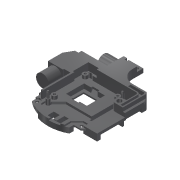
# Autodesk Inventor part: 01_XY_Actuator
Saved by Autodesk Inventor 2019 (Build 230136000, 136)
## iProperties
Created: 2018-09-04
Part Number: 01_XY_Actuator
Material: PC/ABS-Kunststoff
Document SubType Name: Modeling
Designer: Henry John
Density: 0.357273 g/cm^3
Appearance: Glatt - mittelgrau
Author: Henry John
Autodesk Inventor part; units mm, degrees
ref_plane "YZ Plane" through (0, 0, 0) normal (1, 0, 0) x (0, 1, 0)
ref_plane "XZ Plane" through (0, 0, 0) normal (0, 1, 0) x (-1, 0, 0)
ref_plane "XY Plane" through (0, 0, 0) normal (0, 0, 1) x (1, 0, 0)
sketch "Skizze1" plane through (0, 0, 0) normal (0, 0, 1) x (1, 0, 0)
  line L0 (-4.75, -3.625) -> (4.75, -3.625)
  line L1 (4.75, -3.625) -> (4.75, 3.625)
  line L2 (4.75, 3.625) -> (-4.75, 3.625)
  line L3 (-4.75, 3.625) -> (-4.75, -3.625)
  line L4 (-4.75, -3.625) -> (4.75, 3.625) construction
  line L5 (4.75, -3.625) -> (-4.75, 3.625) construction
  line L6 (13.75, -12.125) -> (13.75, 3.475)
  arc A0 (15.75, 5.475) -> (13.75, 3.475) centre (15.75, 3.475) ccw
  arc A1 (16.85, 5.475) -> (17.85, 6.475) centre (16.85, 6.475) ccw
  line L7 (17.85, 6.475) -> (17.85, 12.475)
  line L8 (17.85, 12.475) -> (19.45, 12.475)
  arc A2 (20.45, 11.475) -> (19.45, 12.475) centre (19.45, 11.475) ccw
  line L9 (20.45, 11.475) -> (20.45, 5.475)
  arc A3 (19.95, 4.975) -> (20.45, 5.475) centre (19.95, 5.475) ccw
  line L10 (19.95, 4.975) -> (18.7, 4.975)
  arc A4 (18.7, 4.975) -> (16.25, 2.525) centre (18.7, 2.525) ccw
  line L11 (16.25, 2.525) -> (16.25, -12.525)
  circle A5 centre (18.7, 2.525) radius 1.45
  line L12 (16.25, -12.525) -> (5.5, -12.525)
  line L13 (5.5, -12.525) -> (5.5, -12.125)
  line L14 (5.5, -12.125) -> (13.75, -12.125)
  circle A6 centre (-12.15, -18.0941) radius 0.9
  circle A7 centre (14.85, -17.225) radius 0.9
  line L15 (11.75, -19.125) -> (16.2, -19.125)
  line L16 (16.2, -19.125) -> (17.85, -17.475)
  line L17 (17.85, -17.475) -> (24.75, -17.475)
  line L18 (24.75, -17.475) -> (24.75, 12.025)
  line L19 (24.75, 12.025) -> (22.5561, 15.825)
  line L20 (22.5561, 15.825) -> (13.55, 15.825)
  line L21 (11.75, -19.125) -> (11.75, -21.875)
  line L22 (-14.25, -19.125) -> (-14.25, -13.625)
  line L23 (-15.45, -6.175) -> (-25.25, -6.175)
  line L24 (-25.25, -6.175) -> (-25.25, 10.825)
  line L25 (-25.25, 10.825) -> (-22.3632, 15.825)
  line L26 (-22.3632, 15.825) -> (-20.25, 15.825)
  line L27 (-12.25, 17.825) -> (-12.25, 28.125)
  line L28 (-12.25, 28.125) -> (-3.55, 28.125)
  line L29 (-3.55, 28.125) -> (-3.55, 30.625)
  line L30 (-3.55, 30.625) -> (5.55, 30.625)
  line L31 (5.55, 30.625) -> (5.55, 23.825)
  arc A8 (5.55, 23.825) -> (13.55, 15.825) centre (13.55, 23.825) ccw
  circle A9 centre (3.55, 28.625) radius 0.9
  line L32 (-20.25, 15.825) -> (-20.25, 17.825)
  line L33 (-20.25, 17.825) -> (-12.25, 17.825)
  line L34 (-14.25, -13.625) -> (-15.45, -13.625)
  line L35 (-15.45, -13.625) -> (-15.45, -6.175)
  line L36 (15.75, 5.475) -> (16.85, 5.475)
  arc A10 (-14.25, -19.125) -> (11.75, -21.875) centre (0.8733, -0.4247) ccw
  line L37 (30.6655, -24.475) -> (-37.4601, -24.475) construction
  point P0 (0, 0)
  dimension "d0" = 9.5
  dimension "d1" = 7.25
  dimension "d2" = 9
  dimension "d3" = 2
  dimension "d4" = 1
  dimension "d5" = 6
  dimension "d6" = 2.9
  dimension "d7" = 1
  dimension "d8" = 2.6
  dimension "d9" = 2.5
  dimension "d10" = 7.5
  dimension "d11" = 18
  dimension "d12" = 0.4
  dimension "d15" = 8.5
  dimension "d16" = 1.8
  dimension "d17" = 1.8
  dimension "d18" = 27
  dimension "d19" = 135
  dimension "d20" = 150
  dimension "d21" = 6.6
  dimension "d23" = 1.8
  dimension "d24" = 2
  dimension "d25" = 2
  dimension "d26" = 8
  dimension "d27" = 27
  dimension "d28" = 14.8
  dimension "d30" = 9.1
  dimension "d31" = 17.8
  dimension "d32" = 2.5
  dimension "d33" = 1
  dimension "d34" = 0.5
  dimension "d35" = 2.75
  dimension "d36" = 20
  dimension "d38" = 26
  dimension "d40" = 1.2
  dimension "d41" = 1
  dimension "d42" = 3
  dimension "d44" = 20
  dimension "d46" = 5.5
  dimension "d47" = 1.2
  dimension "d48" = 11
  dimension "d49" = 150
  dimension "d50" = 5
  dimension "d51" = 8
  dimension "d52" = 2
  dimension "d53" = 5
  dimension "d111" = 4.3
  dimension "d221" = 10.75
  dimension "d252" = 50
  dimension "d254" = 55.1
  dimension "d255" = 1.2
  dimension "d256" = 24
  dimension "d269" = 29.5
  constraints: 77 end point, 17 perpendicular, 14 point on circle, 13 tangent, 11 centre point, 6 parallel, 5 horizontal, 4 vertical, 2 midpoint, 1 coincident, 1 collinear, 1 point on line
  measures "d0" distance of L2.end L1.end
  measures "d1" distance of L1.end L0.end
  measures "d2" distance between parallel lines of L6 L1
  measures "d3" radius of A0
  measures "d4" radius of A1
  measures "d5" distance of L7.start L7.end
  measures "d6" diameter of A5
  measures "d7" radial gap between concentric circles of A4 A5
  measures "d8" distance between parallel lines of L9 L7
  measures "d9" distance between parallel lines of L6 L11
  measures "d10" distance between parallel lines of L8 L10
  measures "d11" distance from line of L12 L36.end
  measures "d12" distance between parallel lines of L14 L12
  measures "d15" distance between parallel lines of L14 L0
  measures "d16" diameter of A7
  measures "d17" diameter of A6
  measures "d18" horizontal distance of A7.centre A6.centre
  measures "d19" angle of L16 L15
  measures "d20" angle of L19 L18
  measures "d21" distance between parallel lines of L15 L12
  measures "d23" diameter of A9
  measures "d24" distance from line of A9.centre L30
  measures "d25" distance from line of L31 A9.centre
  measures "d26" radius of A8
  measures "d27" distance between parallel lines of L30 L2
  measures "d28" distance between parallel lines of L20 L30
  measures "d30" distance of L29.end L30.end
  measures "d31" distance between parallel lines of L27 L31
  measures "d32" distance of L28.end L29.end
  measures "d33" radius of A2
  measures "d34" radius of A3
  measures "d35" distance of L15.start L21.end
  measures "d36" distance from line of L17 A4.centre
  measures "d38" distance between parallel lines of L21 L22
  measures "d40" distance edge to line of A6 L22
  measures "d41" distance edge to line of A7 L15
  measures "d42" horizontal distance of A7.centre L16.end
  measures "d44" distance between parallel lines of L18 L1
  measures "d46" distance from line of L22.start L34
  measures "d47" distance between parallel lines of L35 L22
  measures "d48" distance between parallel lines of L24 L22
  measures "d49" angle of L24 L25
  measures "d50" distance from line of L24.end L26
  measures "d51" distance between parallel lines of L32 L27
  measures "d52" distance between parallel lines of L26 L33
  measures "d53" distance between parallel lines of L24 L32
  measures "d111" distance between parallel lines of L18 L9
  measures "d221" distance between parallel lines of L11 L13
  measures "d252" distance between parallel lines of L18 L24
  measures "d256" distance between parallel lines of L23 L33
  measures "d269" distance from line of L18.end L17
extrude "Extrusion1" add sketch "Skizze1" along normal blind 9
sketch "Skizze2" plane through (-25.25, -6.175, 0) normal (0, -1, 0) x (1, 0, 0)
  line L0 (0, 0) -> (9.8, 0) projected
  line L1 (9.8, 0) -> (9.8, 9) projected
  line L2 (0, 9) -> (9.8, 9) projected
  line L3 (0, 0) -> (0, 9) projected
  circle A0 centre (4.5, 4.5) radius 4.5 construction
  circle A1 centre (4.5, 4.5) radius 4
  point P0 (25.25, 0)
  dimension "d60" = 8
  constraints: 3 tangent, 2 centre point, 1 coincident
  measures "d60" diameter of A1
extrude "Extrusion2" cut sketch "Skizze2" against normal blind 8
sketch "Skizze3" plane through (-12.25, 17.825, 0) normal (-1, 0, 0) x (0, 0, 1)
  line L0 (0, 10.3) -> (0, 0) projected
  line L1 (0, 0) -> (9, 0) projected
  line L2 (9, 10.3) -> (9, 0) projected
  line L3 (0, 10.3) -> (9, 10.3) projected
  circle A0 centre (4.5, 5.8) radius 4.5 construction
  circle A1 centre (4.5, 5.8) radius 4
  point P0 (0, -17.825)
  dimension "d61" = 8
  constraints: 3 tangent, 2 centre point, 1 coincident
  measures "d61" diameter of A1
extrude "Extrusion3" cut sketch "Skizze3" against normal blind 8
sketch "Skizze4" plane through (0, 0, 9) normal (0, 0, 1) x (1, 0, 0)
  line L0 (-15.95, 2.525) -> (-11.95, 2.525)
  line L1 (-11.95, 2.525) -> (-11.95, -15.975)
  line L2 (-11.95, -15.975) -> (-10.95, -15.975)
  line L3 (-10.95, -15.975) -> (-10.95, 4.025)
  line L4 (-10.95, 4.025) -> (-11.95, 4.025)
  line L5 (-11.95, 4.025) -> (-11.95, 13.775)
  line L6 (-11.95, 13.775) -> (-5.45, 13.775)
  line L7 (-5.45, 13.775) -> (-5.45, 12.475)
  line L8 (-5.45, 12.475) -> (18.95, 12.475)
  line L9 (20.45, 10.975) -> (20.45, 6.725)
  arc A0 (18.7, 4.975) -> (20.45, 6.725) centre (18.7, 6.725) ccw
  arc A1 (18.7, 4.975) -> (16.25, 2.525) centre (18.7, 2.525) ccw
  line L10 (18.25, -0.025) -> (25.25, -0.025)
  line L11 (25.25, -0.025) -> (25.25, -25.475)
  line L12 (25.25, -25.475) -> (-15.95, -25.475)
  line L13 (-15.95, -25.475) -> (-15.95, 2.525)
  circle A2 centre (18.7, 2.525) radius 1.45 construction
  line L14 (20.45, 11.475) -> (20.45, 5.475) construction
  arc A3 (20.45, 10.975) -> (18.95, 12.475) centre (18.95, 10.975) ccw
  line L15 (17.85, 12.475) -> (19.45, 12.475) projected
  line L16 (-15.45, 1.825) -> (-15.45, -13.625) construction
  line L17 (24.75, -17.475) -> (24.75, 12.025) construction
  arc A4 (18.7, 4.975) -> (16.25, 2.525) centre (18.7, 2.525) ccw construction
  line L18 (16.25, 2.525) -> (16.25, 1.975)
  line L19 (16.25, 2.525) -> (16.25, -12.525) construction
  arc A5 (16.25, 1.975) -> (18.25, -0.025) centre (18.25, 1.975) ccw
  arc A6 (-14.25, -19.125) -> (11.75, -21.875) centre (0.8733, -0.4247) ccw construction
  point P0 (0, 0)
  dimension "d64" = 1.5
  dimension "d66" = 1.3
  dimension "d67" = 6.5
  dimension "d68" = 1
  dimension "d69" = 9.75
  dimension "d70" = 20
  dimension "d71" = 1
  dimension "d72" = 18.5
  dimension "d73" = 0.5
  dimension "d74" = 0.5
  dimension "d75" = 2
  dimension "d76" = 5
  dimension "d257" = 1
  dimension "d258" = 32.4
  constraints: 30 end point, 11 perpendicular, 8 point on circle, 4 centre point, 4 tangent, 2 collinear, 2 horizontal, 2 horizontal alignment, 2 point on line, 2 vertical alignment, 1 coincident, 1 concentric
  measures "d64" radius of A3
  measures "d66" distance between parallel lines of L8 L6
  measures "d67" distance of L5.end L6.end
  measures "d68" distance between parallel lines of L5 L3
  measures "d69" distance between parallel lines of L4 L6
  measures "d70" distance of L2.end L3.end
  measures "d71" distance of L1.end L2.end
  measures "d72" distance of L0.end L1.end
  measures "d73" distance between parallel lines of L16 L13
  measures "d74" distance between parallel lines of L17 L11
  measures "d75" radius of A5
  measures "d76" distance from line of A0.start L10
  measures "d257" distance edge to line of A6 L12
  measures "d258" distance between parallel lines of L5 L9
extrude "Extrusion4" cut sketch "Skizze4" against normal blind 4.7
sketch "Skizze5" plane through (0, 0, 4.3) normal (0, 0, 1) x (1, 0, 0)
  circle A0 centre (-12.15, -18.0941) radius 0.9 projected
  line L0 (-14.25, -13.625) -> (-14.25, -19.125) projected
  line L1 (-14.25, -16.8941) -> (-13.75, -16.8941)
  line L2 (-10.15, -18.0941) -> (-10.15, -21.8)
  line L3 (-10.15, -21.8) -> (-14.25, -21.8)
  line L4 (-14.25, -21.8) -> (-14.25, -16.8941)
  arc A1 (-10.15, -18.0941) -> (-13.75, -16.8941) centre (-12.15, -18.0941) ccw
  line L5 (9.75, -22.7769) -> (9.75, -18.7769)
  line L6 (9.75, -18.7769) -> (13.5519, -14.975)
  line L7 (13.5519, -14.975) -> (16.5519, -14.975)
  line L8 (16.5519, -14.975) -> (16.5519, -17.475)
  line L9 (16.5519, -17.475) -> (18.35, -17.475)
  line L10 (18.35, -17.475) -> (18.35, -22.7769)
  line L11 (18.35, -22.7769) -> (9.75, -22.7769)
  line L12 (24.75, -17.475) -> (17.85, -17.475) construction
  line L13 (11.75, -19.125) -> (11.75, -21.875) construction
  line L14 (7.75, -24.4681) -> (7.75, -16.8171)
  line L15 (7.75, -16.8171) -> (12.4421, -12.125)
  line L16 (13.75, -12.125) -> (13.75, -9.925)
  line L17 (13.75, 3.475) -> (13.75, -12.125) construction
  line L18 (13.75, -9.925) -> (-2.25, -9.925)
  line L19 (-4.75, -3.625) -> (4.75, -3.625) projected
  line L20 (-2.25, -9.925) -> (-6.7793, -14.4543)
  line L21 (-6.7793, -14.4543) -> (-6.7793, -15.4543)
  arc A2 (-9.15, -15.7181) -> (-6.7793, -15.4543) centre (-7.9793, -15.4543) ccw
  line L22 (-9.15, -15.7181) -> (-9.15, -18.4681)
  line L23 (-9.15, -18.4681) -> (-5.55, -22.0681)
  line L24 (-5.55, -22.0681) -> (-3.55, -22.0681)
  line L25 (-3.55, -22.0681) -> (-3.05, -22.5681)
  line L26 (-3.05, -22.5681) -> (-1.05, -22.5681)
  line L27 (-1.05, -22.5681) -> (-0.55, -23.0681)
  line L28 (-0.55, -23.0681) -> (1.45, -23.0681)
  line L29 (1.45, -23.0681) -> (1.45, -24.4681)
  line L30 (1.45, -24.4681) -> (7.75, -24.4681)
  line L31 (5.5, -12.525) -> (16.25, -12.525) construction
  arc A3 (-14.25, -19.125) -> (11.75, -21.875) centre (0.8733, -0.4247) ccw construction
  arc A4 (-14.25, -19.125) -> (11.75, -21.875) centre (0.8733, -0.4247) ccw construction
  line L32 (13.75, -12.125) -> (5.5, -12.125) projected
  line L33 (13.75, -12.125) -> (12.4421, -12.125)
  point P0 (0, 0)
  point P1 (0.2761, -24.4676)
  point P2 (1.4706, -24.4676)
  dimension "d79" = 2
  dimension "d80" = 0.5
  dimension "d81" = 4
  dimension "d82" = 135
  dimension "d83" = 2.5
  dimension "d84" = 3
  dimension "d85" = 2
  dimension "d86" = 0.5
  dimension "d87" = 2.6
  dimension "d90" = 2
  dimension "d91" = 6.3
  dimension "d92" = 1.4
  dimension "d93" = 2
  dimension "d94" = 0.5
  dimension "d95" = 2
  dimension "d96" = 0.5
  dimension "d97" = 2
  dimension "d98" = 1
  dimension "d99" = 1.2
  dimension "d100" = 1
  dimension "d104" = 2.75
  dimension "d105" = 16
  dimension "d280" = 2.8
  constraints: 54 end point, 8 parallel, 7 perpendicular, 7 point on circle, 5 horizontal, 4 collinear, 3 vertical, 2 centre point, 2 point on line, 2 tangent, 1 coincident
  measures "d79" radius of A1
  measures "d80" distance of L1.start L1.end
  measures "d81" distance of L5.start L5.end
  measures "d82" angle of L5 L6
  measures "d83" distance of L7.end L8.end
  measures "d84" distance of L6.end L7.end
  measures "d85" distance between parallel lines of L13 L5
  measures "d86" distance from line of L12.end L10
  measures "d87" distance between parallel lines of L31 L18
  measures "d90" distance between parallel lines of L14 L5
  measures "d91" distance between parallel lines of L29 L14
  measures "d92" distance of L28.end L29.end
  measures "d93" distance of L27.end L28.end
  measures "d94" distance between parallel lines of L26 L28
  measures "d95" distance of L25.end L26.end
  measures "d96" distance between parallel lines of L26 L24
  measures "d97" distance of L23.end L24.end
  measures "d98" distance between parallel lines of L22 L2
  measures "d99" radius of A2
  measures "d100" distance of L20.end L21.end
  measures "d104" distance of L22.start L22.end
  measures "d105" distance of L16.end L18.end
  measures "d280" distance between parallel lines of L6 L15
extrude "Extrusion5" cut sketch "Skizze5" against normal blind 1
sketch "Skizze6" plane through (0, 0, 9) normal (0, 0, 1) x (1, 0, 0)
  line L0 (23.35, 14.4499) -> (24.75, 14.4499)
  line L1 (24.75, 14.4499) -> (24.75, -0.025)
  line L2 (24.75, -0.025) -> (23.35, -0.025)
  line L3 (23.35, -0.025) -> (23.35, 14.4499)
  line L4 (20.45, 11.475) -> (20.45, 5.475) construction
  line L5 (24.75, -0.025) -> (24.75, 12.025) construction
  line L6 (24.75, 12.025) -> (22.5561, 15.825) construction
  line L7 (18.25, -0.025) -> (24.75, -0.025) construction
  line L8 (21.15, 0.775) -> (22.55, 0.775)
  line L9 (22.55, 0.775) -> (22.55, 13.8355)
  line L10 (22.55, 13.8355) -> (21.9787, 14.825)
  line L11 (21.9787, 14.825) -> (13.45, 14.825)
  line L12 (13.45, 14.825) -> (13.45, 13.175)
  line L13 (13.45, 13.175) -> (19.45, 13.175)
  arc A0 (21.15, 11.475) -> (19.45, 13.175) centre (19.45, 11.475) ccw
  line L14 (21.15, 11.475) -> (21.15, 0.775)
  arc A1 (20.45, 11.475) -> (19.45, 12.475) centre (19.45, 11.475) ccw construction
  circle A2 centre (18.7, 2.525) radius 1.45 construction
  line L15 (22.5561, 15.825) -> (13.55, 15.825) construction
  point P0 (0, 0)
  dimension "d110" = 2.9
  dimension "d112" = 0.8
  dimension "d113" = 1
  dimension "d114" = 1
  dimension "d115" = 1
  dimension "d116" = 0.8
  dimension "d117" = 7
  constraints: 22 end point, 4 parallel, 4 perpendicular, 2 collinear, 2 horizontal, 2 point on circle, 2 tangent, 1 centre point, 1 concentric, 1 point on line, 1 vertical
  measures "d110" distance between parallel lines of L4 L3
  measures "d112" distance between parallel lines of L7 L8
  measures "d113" distance edge to line of A2 L14
  measures "d114" distance between parallel lines of L15 L11
  measures "d115" distance between parallel lines of L6 L10
  measures "d116" distance between parallel lines of L3 L9
  measures "d117" distance between parallel lines of L12 L4
extrude "Extrusion6" cut sketch "Skizze6" against normal blind 2.3
sketch "Skizze7" plane through (0, 0, 4.3) normal (0, 0, 1) x (1, 0, 0)
  circle A0 centre (-7.9793, -15.4543) radius 1.2
  arc A1 (-9.15, -15.7181) -> (-6.7793, -15.4543) centre (-7.9793, -15.4543) ccw construction
  circle A2 centre (-7.9793, -11.4543) radius 1.575
  circle A3 centre (-7.9793, -11.4543) radius 0.7
  circle A4 centre (-9.45, 9.3) radius 1.575
  circle A5 centre (-9.45, 9.3) radius 0.7
  circle A6 centre (12.7, 7.475) radius 1.575
  circle A7 centre (12.7, 7.475) radius 0.7
  line L0 (-5.45, 12.475) -> (19.45, 12.475) construction
  circle A8 centre (15.7, 7.475) radius 0.75
  line L1 (-11.95, 4.025) -> (-11.95, 13.775) projected
  line L2 (20.45, 11.475) -> (20.45, 5.475) construction
  line L3 (-11.95, 13.775) -> (-5.45, 13.775) construction
  point P0 (0, 0)
  dimension "d120" = 3.15
  dimension "d121" = 1.4
  dimension "d122" = 4
  dimension "d123" = 3.15
  dimension "d124" = 1.4
  dimension "d127" = 3.15
  dimension "d128" = 1.4
  dimension "d130" = 5
  dimension "d132" = 1.5
  dimension "d281" = 2.5
  dimension "d282" = 4
  dimension "d283" = 3
  dimension "d284" = 2.9
  constraints: 8 centre point, 3 coincident, 2 concentric, 1 horizontal alignment, 1 vertical alignment
  measures "d120" diameter of A2
  measures "d121" diameter of A3
  measures "d122" distance of A2.centre A0.centre
  measures "d123" diameter of A4
  measures "d124" diameter of A5
  measures "d127" diameter of A6
  measures "d128" diameter of A7
  measures "d130" distance from line of A6.centre L0
  measures "d132" diameter of A8
  measures "d281" distance from line of L1 A4.centre
  measures "d282" distance edge to line of A8 L2
  measures "d283" distance of A8.centre A6.centre
  measures "d284" distance edge to line of A4 L3
extrude "Extrusion7" add sketch "Skizze7" along normal blind 2
sketch "Skizze8" plane through (-7.9793, -15.4543, 6.3) normal (0, 0, 1) x (1, 0, 0)
  circle A0 centre (0, 0) radius 1.2 construction
  circle A1 centre (23.6793, 22.9293) radius 0.75 projected
  circle A2 centre (0, 0) radius 0.75
  point P0 (7.9793, 15.4543)
  dimension "d135" = 1.5
  constraints: 1 centre point, 1 coincident
  measures "d135" diameter of A2
extrude "Extrusion8" add sketch "Skizze8" along normal blind 4
sketch "Skizze9" plane through (0, 0, 9) normal (0, 0, 1) x (1, 0, 0)
  line L0 (-3.55, 30.625) -> (-3.55, 28.125) projected
  line L1 (-3.55, 28.125) -> (-2.05, 28.125)
  line L2 (-2.05, 28.125) -> (-2.05, 26.625)
  line L3 (-2.05, 26.625) -> (5.55, 26.625)
  line L4 (5.55, 26.625) -> (5.55, 30.625)
  line L5 (5.55, 30.625) -> (-3.55, 30.625) projected
  line L6 (5.55, 30.625) -> (-3.55, 30.625)
  line L7 (-3.55, 30.625) -> (-3.55, 28.125)
  point P0 (0, 0)
  dimension "d138" = 1.5
  constraints: 12 end point, 5 perpendicular, 1 collinear, 1 horizontal
  measures "d138" distance of L0.end L1.end
extrude "Extrusion9" cut sketch "Skizze9" against normal blind 3
sketch "Skizze10" plane through (0, 0, 0) normal (0, 0, -1) x (-1, 0, 0)
  line L0 (2.05, 26.625) -> (2.05, 28.125) projected
  line L1 (2.05, 28.125) -> (3.55, 28.125) projected
  line L2 (3.55, 28.125) -> (3.55, 30.625) projected
  line L3 (3.55, 30.625) -> (-5.55, 30.625) projected
  line L4 (2.05, 26.625) -> (2.05, 15.925)
  line L5 (2.05, 15.925) -> (1.55, 15.925)
  line L6 (0.55, 18.925) -> (0.55, 24.625)
  line L7 (0.55, 24.625) -> (-2.45, 24.625)
  line L8 (-2.45, 24.625) -> (-2.45, 19.625)
  line L9 (-2.45, 19.625) -> (-3.45, 19.625)
  arc A0 (-8.55, 15.825) -> (-3.45, 19.625) centre (-10.386, 23.6115) ccw
  line L10 (-8.55, 15.825) -> (-13.55, 15.825)
  arc A1 (-13.55, 15.825) -> (-5.55, 23.825) centre (-13.55, 23.825) ccw projected
  arc A2 (-13.55, 15.825) -> (-5.55, 23.825) centre (-13.55, 23.825) ccw projected
  line L11 (-5.55, 23.825) -> (-5.55, 30.625) projected
  arc A3 (-13.55, 15.825) -> (-5.55, 23.825) centre (-13.55, 23.825) ccw projected
  line L12 (-0.45, 23.625) -> (-1.45, 23.625)
  line L13 (-1.45, 23.625) -> (-1.45, 18.625)
  line L14 (-1.45, 18.625) -> (-2.8937, 18.625)
  arc A4 (-5.7043, 15.925) -> (-2.8937, 18.625) centre (-10.386, 23.6115) ccw
  line L15 (-5.7043, 15.925) -> (0.4959, 15.925)
  line L16 (0.4959, 15.925) -> (-0.45, 18.7627)
  line L17 (-0.45, 18.7627) -> (-0.45, 23.625)
  line L18 (1.55, 15.925) -> (0.55, 18.925)
  point P0 (0, 0)
  dimension "d141" = 5
  dimension "d142" = 1
  dimension "d143" = 3
  dimension "d144" = 1.5
  dimension "d145" = 14.7
  dimension "d146" = 6
  dimension "d147" = 11
  dimension "d148" = 3
  dimension "d149" = 1
  dimension "d150" = 1
  dimension "d151" = 1
  dimension "d152" = 1
  dimension "d153" = 1
  dimension "d154" = 1
  dimension "d155" = 1
  constraints: 28 end point, 7 perpendicular, 5 point on circle, 3 horizontal, 2 centre point, 2 vertical, 1 collinear, 1 concentric, 1 equal radius, 1 parallel
  measures "d141" distance of L10.start L10.end
  measures "d142" distance of L8.end L9.end
  measures "d143" distance of L6.end L7.end
  measures "d144" distance between parallel lines of L4 L6
  measures "d145" distance between parallel lines of L3 L5
  measures "d146" distance between parallel lines of L3 L7
  measures "d147" distance between parallel lines of L9 L3
  measures "d148" distance from line of L6.start L5
  measures "d149" distance from line of L5.end L6
  measures "d150" distance between parallel lines of L17 L6
  measures "d151" distance between parallel lines of L8 L13
  measures "d152" distance between parallel lines of L7 L12
  measures "d153" distance between parallel lines of L18 L16
  measures "d154" radial gap between concentric circles of A0 A4
  measures "d155" distance between parallel lines of L9 L14
extrude "Extrusion10" cut sketch "Skizze10" against normal blind 3.5
sketch "Skizze12" plane through (0, 0, 0) normal (0, 0, -1) x (-1, 0, 0)
  line L0 (-17.85, -17.475) -> (-16.2, -17.475)
  line L1 (-16.2, -17.475) -> (-16.2, -14.125)
  line L2 (-16.2, -14.125) -> (-7.6, -14.125)
  line L3 (-7.6, -14.125) -> (-7.6, -19.125)
  line L4 (-7.6, -19.125) -> (-16.2, -19.125)
  line L5 (-16.2, -19.125) -> (-17.85, -17.475)
  circle A0 centre (-9.6, -16.625) radius 0.75
  point P0 (0, 0)
  dimension "d165" = 5
  dimension "d166" = 8.6
  dimension "d167" = 1.5
  dimension "d168" = 2.5
  dimension "d169" = 2
  constraints: 12 end point, 4 perpendicular, 2 coincident, 1 centre point, 1 horizontal, 1 point on line
  measures "d165" distance between parallel lines of L4 L2
  measures "d166" distance between parallel lines of L3 L1
  measures "d167" diameter of A0
  measures "d168" distance from line of A0.centre L4
  measures "d169" distance from line of L3 A0.centre
extrude "Extrusion12" cut sketch "Skizze12" against normal blind 2.5
chamfer "Fase1" distance 0.25 distance2 1 1 edges at (10.35, -16.625, 0) measured on face at (9.85, -16.625, 0)
chamfer "Fase2" distance 0.25 distance2 1 1 edges at (-8.7293, -15.4543, 10.3) measured on face at (-8.2293, -15.4543, 10.3)
chamfer "Fase3" distance 0.25 distance2 1 1 edges at (14.95, 7.475, 10.3) measured on face at (15.45, 7.475, 10.3)
sketch "Skizze11" plane through (0, 0, 0) normal (0, 0, -1) x (-1, 0, 0)
  line L0 (6.45, -23.3329) -> (6.45, -18.125)
  line L1 (6.45, -18.125) -> (9.5, -18.125)
  line L2 (9.5, -18.125) -> (9.5, -14.625)
  line L3 (9.5, -14.625) -> (10.5, -13.625)
  line L4 (10.5, -13.625) -> (15.45, -13.625)
  line L5 (15.45, -13.625) -> (15.45, -23.3329)
  line L6 (15.45, -23.3329) -> (6.45, -23.3329)
  line L7 (15.45, -13.625) -> (14.25, -13.625) construction
  line L8 (15.45, -13.625) -> (15.45, 1.825) construction
  line L9 (14.25, -13.625) -> (14.25, -19.125) projected
  arc A0 (-11.75, -21.875) -> (14.25, -19.125) centre (-0.8733, -0.4247) ccw construction
  point P0 (0, 0)
  dimension "d158" = 135
  dimension "d160" = 1
  dimension "d161" = 4.5
  dimension "d162" = 9
  dimension "d223" = 4.75
  constraints: 14 end point, 3 perpendicular, 2 collinear, 1 horizontal, 1 parallel, 1 point on circle, 1 vertical
  measures "d158" angle of L2 L3
  measures "d160" distance from line of L2.end L4
  measures "d161" distance between parallel lines of L4 L1
  measures "d162" distance between parallel lines of L0 L5
  measures "d223" distance between parallel lines of L2 L9
extrude "Extrusion11" cut sketch "Skizze11" against normal blind 2.3
sketch "Skizze13" plane through (0, 0, 0) normal (0, 0, -1) x (-1, 0, 0)
  line L0 (6.95, 6.15) -> (-3.8, 6.15)
  line L1 (-3.8, 6.15) -> (-3.8, 7.65)
  arc A0 (-3.8, 7.65) -> (-6.2, 7.65) centre (-5, 7.65) ccw
  line L2 (-6.2, 7.65) -> (-6.2, 6.15)
  line L3 (-6.2, 6.15) -> (-6.95, 6.15)
  line L4 (-6.95, 6.15) -> (-6.95, -6.15)
  line L5 (-6.95, -6.15) -> (3.75, -6.15)
  line L6 (3.75, -6.15) -> (3.75, -7.65)
  arc A1 (3.75, -7.65) -> (6.15, -7.65) centre (4.95, -7.65) ccw
  line L7 (6.15, -7.65) -> (6.15, -6.15)
  line L8 (6.15, -6.15) -> (6.95, -6.15)
  line L9 (6.95, -6.15) -> (6.95, 6.15)
  line L10 (3.25, -6.65) -> (3.25, -8.1)
  arc A2 (3.25, -8.1) -> (4.25, -9.1) centre (4.25, -8.1) ccw
  line L11 (4.25, -9.1) -> (6.45, -9.1)
  arc A3 (6.45, -9.1) -> (7.45, -8.1) centre (6.45, -8.1) ccw
  line L12 (7.45, -8.1) -> (7.45, 9.15)
  line L13 (7.45, 9.15) -> (-3.25, 9.15)
  line L14 (-3.25, 9.15) -> (-3.25, 10.65)
  arc A4 (-3.25, 10.65) -> (-4.25, 11.65) centre (-4.25, 10.65) ccw
  line L15 (-4.25, 11.65) -> (-6.75, 11.65)
  arc A5 (-6.75, 11.65) -> (-7.75, 10.65) centre (-6.75, 10.65) ccw
  line L16 (-7.75, 10.65) -> (-7.75, -6.65)
  line L17 (-7.75, -6.65) -> (3.25, -6.65)
  line L18 (6.95, 6.15) -> (-6.95, -6.15) construction
  line L19 (6.95, -6.15) -> (-6.95, 6.15) construction
  circle A6 centre (4.95, -7.65) radius 0.45
  circle A7 centre (-5, 7.65) radius 0.45
  line L20 (1.7, -21.525) -> (1.7, -18.325)
  line L21 (6.45, -18.125) -> (-2.05, -18.125)
  line L22 (-2.05, -18.125) -> (-2.05, -22.125)
  line L23 (-2.05, -22.125) -> (-4.05, -22.125)
  line L24 (-4.05, -22.125) -> (-4.05, -13.575)
  line L25 (-4.05, -13.575) -> (-5.5, -12.125)
  line L26 (-5.5, -12.125) -> (-9.8, -12.125)
  line L27 (-9.8, -12.125) -> (-9.8, -12.525)
  line L28 (-9.8, -12.525) -> (-7.8, -12.525)
  line L29 (-7.8, -12.525) -> (-6.8, -13.525)
  line L30 (-6.8, -13.525) -> (-6.8, -20.025)
  line L31 (-6.8, -20.025) -> (-8.3, -20.025)
  line L32 (-8.3, -20.025) -> (-8.3, -21.525)
  line L33 (-8.3, -21.525) -> (-6.8, -21.525)
  arc A8 (-6.8, -21.525) -> (-5.8, -22.525) centre (-5.8, -21.525) ccw
  line L34 (-5.8, -22.525) -> (0.7, -22.525)
  arc A9 (0.7, -22.525) -> (1.7, -21.525) centre (0.7, -21.525) ccw
  line L35 (-5.5, -12.525) -> (-16.25, -12.525) construction
  line L36 (-13.75, -12.125) -> (-5.5, -12.125) construction
  line L37 (-7.6, -14.125) -> (-7.6, -19.125) construction
  line L38 (-16.25, -12.525) -> (-16.25, 2.525) construction
  line L39 (-7.6, -19.125) -> (-11.75, -19.125) construction
  line L40 (9.5, -18.125) -> (9.5, -14.625) construction
  line L41 (6.45, -18.125) -> (9.5, -18.125) construction
  line L42 (1.7, -18.325) -> (6.45, -18.325)
  line L43 (6.45, -18.325) -> (6.45, -18.125)
  point P0 (0, 0)
  point P1 (0, 0)
  point P2 (0, 0)
  dimension "d181" = 15.2
  dimension "d182" = 15.8
  dimension "d183" = 4.5
  dimension "d184" = 1
  dimension "d185" = 3
  dimension "d186" = 0.5
  dimension "d187" = 2.4
  dimension "d188" = 1.5
  dimension "d189" = 0.8
  dimension "d190" = 0.5
  dimension "d191" = 2
  dimension "d193" = 2.4
  dimension "d195" = 4.2
  dimension "d196" = 18.25
  dimension "d197" = 1.5
  dimension "d198" = 18.3
  dimension "d199" = 2.75
  dimension "d202" = 0.9
  dimension "d203" = 0.9
  dimension "d207" = 0.8
  dimension "d210" = 1
  dimension "d211" = 0.9
  dimension "d212" = 1.5
  dimension "d213" = 1
  dimension "d214" = 8.5
  dimension "d219" = 0.4
  dimension "d224" = 0.2
  dimension "d225" = 45
  dimension "d230" = 1.5
  dimension "d231" = 2
  dimension "d232" = 2.75
  dimension "d233" = 2
  constraints: 74 end point, 22 perpendicular, 16 point on circle, 14 tangent, 10 centre point, 6 point on line, 4 equal radius, 4 horizontal, 3 coincident, 3 parallel, 2 collinear, 2 midpoint, 2 vertical, 1 vertical alignment
  measures "d181" distance between parallel lines of L16 L12
  measures "d182" distance between parallel lines of L13 L17
  measures "d183" distance between parallel lines of L16 L14
  measures "d184" radius of A4
  measures "d185" distance between parallel lines of L13 L0
  measures "d186" distance between parallel lines of L5 L17
  measures "d187" distance between parallel lines of L2 L1
  measures "d188" distance from line of L0 A0.centre
  measures "d189" distance between parallel lines of L16 L4
  measures "d190" distance between parallel lines of L12 L9
  measures "d191" distance from line of L9 A1.centre
  measures "d193" distance between parallel lines of L6 L7
  measures "d195" distance between parallel lines of L10 L12
  measures "d196" distance between parallel lines of L13 L11
  measures "d197" distance from line of L5 A1.centre
  measures "d198" distance between parallel lines of L17 L15
  measures "d199" distance from line of L16 A0.centre
  measures "d202" diameter of A6
  measures "d203" diameter of A7
  measures "d207" distance between parallel lines of L30 L37
  measures "d210" distance from line of L28 L29.end
  measures "d211" distance between parallel lines of L39 L31
  measures "d212" distance of L30.end L31.end
  measures "d213" radius of A8
  measures "d214" distance between parallel lines of L20 L30
  measures "d219" distance between parallel lines of L34 L23
  measures "d224" distance between parallel lines of L21 L42
  measures "d225" angle of L30 L29
  measures "d230" distance between parallel lines of L31 L33
  measures "d231" distance from line of L28.end L27
  measures "d232" distance between parallel lines of L30 L24
  measures "d233" distance between parallel lines of L22 L24
extrude "Extrusion13" cut sketch "Skizze13" against normal blind 2
sketch "Skizze14" plane through (0, 0, 0) normal (0, 0, -1) x (-1, 0, 0)
  line L0 (4.75, 3.625) -> (4.75, -3.625) projected
  line L1 (4.75, -3.625) -> (-4.75, -3.625) projected
  line L2 (-4.75, -3.625) -> (-4.75, 3.625) projected
  line L3 (-4.75, 3.625) -> (4.75, 3.625) projected
  circle A0 centre (-5, 7.65) radius 0.45 projected
  line L4 (-3.8, 6.15) -> (-3.8, 7.65) projected
  arc A1 (-3.8, 7.65) -> (-6.2, 7.65) centre (-5, 7.65) ccw projected
  line L5 (-6.2, 7.65) -> (-6.2, 6.15) projected
  line L6 (-6.2, 6.15) -> (-6.95, 6.15) projected
  line L7 (-6.95, 6.15) -> (-6.95, -6.15) projected
  line L8 (-6.95, -6.15) -> (3.75, -6.15) projected
  line L9 (3.75, -6.15) -> (3.75, -7.65) projected
  arc A2 (3.75, -7.65) -> (6.15, -7.65) centre (4.95, -7.65) ccw projected
  line L10 (6.15, -7.65) -> (6.15, -6.15) projected
  line L11 (6.15, -6.15) -> (6.95, -6.15) projected
  line L12 (6.95, -6.15) -> (6.95, 6.15) projected
  line L13 (6.95, 6.15) -> (-3.8, 6.15) projected
  circle A3 centre (4.95, -7.65) radius 0.45 projected
extrude "Extrusion14" cut sketch "Skizze14" against normal blind 0.5
sketch "Skizze15" plane through (0, 0, 2) normal (0, 0, -1) x (-1, 0, 0)
  arc A0 (-3.25, 10.65) -> (-4.25, 11.65) centre (-4.25, 10.65) ccw projected
  line L0 (-6.75, 11.65) -> (-4.25, 11.65) projected
  arc A1 (-6.75, 11.65) -> (-7.75, 10.65) centre (-6.75, 10.65) ccw projected
  line L1 (-3.25, 9.85) -> (-7.75, 9.85)
  line L2 (-7.75, 10.65) -> (-7.75, 9.85)
  line L3 (-3.25, 10.65) -> (-3.25, 9.85)
  line L4 (1.7, -18.325) -> (1.7, -21.525) projected
  arc A2 (0.7, -22.525) -> (1.7, -21.525) centre (0.7, -21.525) ccw projected
  line L5 (0.7, -22.525) -> (-5.8, -22.525) projected
  arc A3 (-6.8, -21.525) -> (-5.8, -22.525) centre (-5.8, -21.525) ccw projected
  line L6 (-2.05, -22.125) -> (-2.05, -18.125) projected
  line L7 (-4.05, -22.125) -> (-2.05, -22.125) projected
  line L8 (-4.05, -22.125) -> (-4.05, -17.225)
  line L9 (-4.05, -17.225) -> (-6.8, -17.225)
  line L10 (-6.8, -17.225) -> (-6.8, -21.525)
  line L11 (-2.05, -18.125) -> (1.7, -18.125)
  line L12 (1.7, -18.125) -> (1.7, -18.325)
  point P0 (0, 0)
  dimension "d226" = 1.8
  dimension "d227" = 5.3
  constraints: 16 end point, 3 perpendicular, 3 vertical, 2 horizontal
  measures "d226" distance between parallel lines of L0 L1
  measures "d227" distance between parallel lines of L9 L5
extrude "Extrusion15" cut sketch "Skizze15" along normal through all both and the other way through all
sketch "Skizze16" plane through (0, 0, 4.3) normal (0, 0, 1) x (1, 0, 0)
  line L0 (-6.5, 5.625) -> (-6.5, -5.625)
  line L1 (6.5, -5.625) -> (6.5, 5.625)
  line L2 (-2.1, 5.625) -> (-2.1, 6.65)
  line L3 (-2.1, 6.65) -> (2.1, 6.65)
  line L4 (2.1, 6.65) -> (2.1, 5.625)
  line L5 (2.1, -5.625) -> (2.1, -6.65)
  line L6 (2.1, -6.65) -> (-2.1, -6.65)
  line L7 (-2.1, -6.65) -> (-2.1, -5.625)
  line L8 (-6.5, -5.625) -> (-2.1, -5.625)
  line L9 (2.1, -5.625) -> (6.5, -5.625)
  line L10 (6.5, 5.625) -> (2.1, 5.625)
  line L11 (-2.1, 5.625) -> (-6.5, 5.625)
  line L12 (-6.5, -5.625) -> (6.5, 5.625) construction
  line L13 (-6.5, 5.625) -> (6.5, -5.625) construction
  line L14 (-2.1, 6.65) -> (2.1, -6.65) construction
  line L15 (-2.1, -6.65) -> (2.1, 6.65) construction
  point P0 (0, 0)
  point P1 (0, 0)
  point P2 (0, -6.65)
  dimension "d234" = 4.2
  dimension "d235" = 13
  dimension "d236" = 11.25
  dimension "d237" = 13.3
  constraints: 32 end point, 6 perpendicular, 5 parallel, 4 midpoint, 4 point on line, 2 collinear, 2 horizontal, 1 coincident, 1 vertical, 1 vertical alignment
  measures "d234" distance between parallel lines of L7 L5
  measures "d235" distance between parallel lines of L0 L1
  measures "d236" distance between parallel lines of L9 L10
  measures "d237" distance between parallel lines of L6 L3
extrude "Extrusion16" cut sketch "Skizze16" against normal blind 2.9
sketch "Skizze17" plane through (0, 0, 3.3) normal (0, 0, 1) x (1, 0, 0)
  arc A0 (-9.1793, -15.4543) -> (-7.6793, -16.9543) centre (-7.6793, -15.4543) ccw
  arc A1 (-6.4509, -16.9543) -> (-4.9509, -15.4543) centre (-6.4509, -15.4543) ccw
  line L0 (-7.6793, -16.9543) -> (-6.4509, -16.9543)
  line L1 (-4.9509, -15.4543) -> (-2.0216, -12.525)
  line L2 (-2.0216, -12.525) -> (13.75, -12.525)
  line L3 (13.75, -9.925) -> (-2.25, -9.925)
  line L4 (-2.25, -9.925) -> (-6.7793, -14.4543)
  line L5 (-6.7793, -14.4543) -> (-6.7793, -15.4543)
  line L6 (-2.25, -9.925) -> (13.75, -9.925) construction
  line L7 (5.5, -12.525) -> (12.0421, -12.525) construction
  line L8 (-6.7793, -14.4543) -> (-2.25, -9.925) construction
  line L9 (-6.7793, -15.4543) -> (-6.7793, -14.4543) construction
  circle A2 centre (-7.9793, -15.4543) radius 1.2 construction
  arc A3 (-9.1793, -15.4543) -> (-6.7793, -15.4543) centre (-7.9793, -15.4543) ccw
  line L10 (13.75, -9.925) -> (13.75, -12.525)
  line L11 (13.75, 3.475) -> (13.75, -12.125) construction
  point P0 (0, 0)
  point P1 (13.5714, -9.925)
  dimension "d241" = 1.5
  dimension "d243" = 2
  constraints: 14 end point, 7 point on circle, 4 collinear, 4 horizontal alignment, 4 point on line, 3 centre point, 3 tangent, 2 horizontal, 1 concentric, 1 parallel, 1 perpendicular
  measures "d241" radius of A1
  measures "d243" distance between parallel lines of L1 L4
extrude "Extrusion17" cut sketch "Skizze17" against normal blind 0.4
sketch "Skizze18" plane through (0, 0, 4.3) normal (0, 0, 1) x (1, 0, 0)
  line L0 (7.75, 9.85) -> (3.25, 9.85) projected
  line L1 (7.75, 9.85) -> (15.85, 9.85)
  arc A0 (17.85, 7.85) -> (15.85, 9.85) centre (15.85, 7.85) ccw
  line L2 (17.85, 12.475) -> (17.85, 6.475) construction
  line L3 (17.85, 7.85) -> (17.85, 6.475)
  line L4 (17.85, 6.475) -> (18.85, 6.475)
  line L5 (18.85, 6.475) -> (18.85, 12.475)
  line L6 (18.85, 12.475) -> (-5.45, 12.475)
  line L7 (-5.45, 12.475) -> (-7.95, 12.475)
  line L8 (3.25, 9.85) -> (-7.9742, 9.85)
  circle A1 centre (-9.45, 9.3) radius 1.575 construction
  line L9 (-11.95, 10.875) -> (-11.95, 12.375)
  arc A2 (-7.95, 12.475) -> (-11.95, 12.375) centre (-9.9155, 11.0435) ccw
  line L10 (20.45, 5.475) -> (20.45, 11.475) construction
  arc A3 (-7.9742, 9.85) -> (-9.45, 10.875) centre (-9.45, 9.3) ccw
  line L11 (-9.45, 10.875) -> (-11.95, 10.875)
  line L12 (-5.45, 13.775) -> (-5.45, 12.475) construction
  point P0 (0, 0)
  dimension "d246" = 1
  dimension "d247" = 2
  dimension "d248" = 1
  dimension "d251" = 32.4
  dimension "d285" = 1.5
  dimension "d287" = 2.5
  constraints: 18 end point, 6 point on circle, 4 horizontal, 3 centre point, 3 tangent, 2 perpendicular, 2 point on line, 1 coincident, 1 collinear, 3 other
  measures "d246" distance from line of L3.start L5
  measures "d247" radius of A0
  measures "d248" distance edge to line of A2 L7
  measures "d251" distance between parallel lines of L9 L10
  measures "d285" distance from line of L9.end L11
  measures "d287" distance of L6.end L7.end
extrude "Extrusion18" cut sketch "Skizze18" against normal blind 3
sketch "Skizze19" plane through (0, 0, 0) normal (0, 0, -1) x (-1, 0, 0)
  line L0 (-24.75, -1.675) -> (-17.85, -1.675)
  line L1 (-17.85, -1.675) -> (-17.85, -15.275)
  line L2 (-17.85, -15.275) -> (-24.75, -15.275)
  line L3 (-24.75, -15.275) -> (-24.75, -1.675)
  line L4 (-24.75, -17.475) -> (-24.75, 12.025) construction
  line L5 (-24.75, -17.475) -> (-16.2, -17.475) projected
  line L6 (-16.25, -12.525) -> (-16.25, 2.525) construction
  line L7 (-24.75, 12.025) -> (-21.65, 12.025)
  line L8 (-21.65, 12.025) -> (-21.65, -0.675)
  line L9 (-21.65, -0.675) -> (-24.75, -0.675)
  line L10 (-24.75, -0.675) -> (-24.75, 12.025)
  line L11 (-20.45, 5.475) -> (-20.45, 11.475) construction
  point P0 (0, 0)
  dimension "d262" = 2.2
  dimension "d263" = 1.6
  dimension "d264" = 1.2
  dimension "d265" = 1
  dimension "d268" = 13.6
  constraints: 16 end point, 4 parallel, 2 collinear, 2 horizontal, 2 perpendicular, 1 point on line
  measures "d262" distance between parallel lines of L2 L5
  measures "d263" distance between parallel lines of L1 L6
  measures "d264" distance between parallel lines of L11 L8
  measures "d265" distance between parallel lines of L0 L9
  measures "d268" distance between parallel lines of L2 L0
extrude "Extrusion19" cut sketch "Skizze19" against normal blind 2.6
sketch "Skizze20" plane through (0, 0, 0) normal (0, 0, -1) x (-1, 0, 0)
  line L0 (-24.75, -0.025) -> (-23.35, -0.025) construction
  line L1 (-18.25, -0.025) -> (-23.35, -0.025) construction
  line L2 (-18.25, -0.025) -> (-24.75, -0.025) construction
  line L3 (-24.75, -0.675) -> (-24.75, 12.025) construction
  line L4 (-21.65, 12.025) -> (-21.65, -0.675) construction
  line L5 (-24.75, 12.025) -> (-21.65, 12.025) construction
  line L6 (-24.75, 0.575) -> (-23.25, 0.575)
  line L7 (-23.25, 0.575) -> (-23.25, 15.825)
  line L8 (-23.25, 15.825) -> (-24.75, 15.825)
  line L9 (-24.75, 15.825) -> (-24.75, 0.575)
  line L10 (-24.75, -1.675) -> (-17.85, -1.675) construction
  point P0 (0, 0)
  point P1 (-22.5561, 15.825)
  dimension "d272" = 1.6
  dimension "d273" = 2.25
  constraints: 8 end point, 2 parallel, 2 point on line, 1 horizontal, 1 perpendicular
  measures "d272" distance between parallel lines of L7 L4
  measures "d273" distance between parallel lines of L6 L10
extrude "Extrusion20" cut sketch "Skizze20" against normal blind 5
ref_plane "Arbeitsebene1" through (-2.6, 5.625, 4.3) normal (1, 0, 0) x (0, 0, -1)
sketch "Skizze21" plane through (-2.6, 5.625, 4.3) normal (1, 0, 0) x (0, 0, -1)
  line L0 (0, 1.025) -> (2.3, 1.025) construction
  line L1 (3.8, 0.525) -> (2.3, 1.025)
  line L2 (2.9, 0) -> (1.15, 1.025)
  line L3 (2.9, 0) -> (3.8, 0.525)
  line L4 (1.15, 1.025) -> (2.3, 1.025)
  line L5 (-5.7, -5.625) -> (4.3, -5.625) construction
  line L6 (0, -12.275) -> (2.3, -12.275) construction
  line L7 (3.8, -11.775) -> (2.3, -12.275)
  line L8 (2.9, -11.25) -> (1.15, -12.275)
  line L9 (2.9, -11.25) -> (3.8, -11.775)
  line L10 (1.15, -12.275) -> (2.3, -12.275)
  point P0 (4.3, -5.625)
  dimension "d279" = 10
  constraints: 20 end point, 5 symmetric about line, 3 midpoint, 1 coincident, 1 collinear, 1 horizontal
  measures "d279" distance of L5.start L5.end
extrude "Extrusion21" add sketch "Skizze21" along normal blind 6
equation "\"d17\" = d16"
